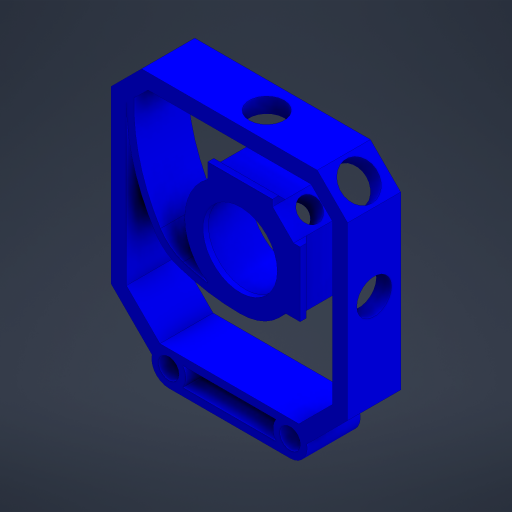
# Autodesk Inventor part: Half Inch Lense Holder (V5)
Saved by Autodesk Inventor 2023.4 (Build 274418000, 418)
## iProperties
Created: 2022-07-25
Part Number: Half Inch Lense Holder (V5)
Material: Generic
Document SubType Name: Modeling
Designer: xSibe
Density: 1 g/cm^3
Appearance: Plastic Blue
Author: xSibe
Autodesk Inventor part; units mm, degrees
ref_plane "YZ Plane" through (0, 0, 0) normal (1, 0, 0) x (0, 1, 0)
ref_plane "XZ Plane" through (0, 0, 0) normal (0, 1, 0) x (-1, 0, 0)
sketch "Sketch1" plane through (0, 0, 0) normal (0, 0, 1) x (1, 0, 0)
  circle A0 centre (10, 3.85) radius 1.5625 projected
  circle A1 centre (-10, 3.85) radius 1.5625 projected
  line L0 (-16.9, 0) -> (16.9, 0) projected
  line L1 (16.9, 0) -> (16.9, 7.7) projected
  line L2 (-16.9, 7.7) -> (16.9, 7.7) projected
  line L3 (-16.9, 0) -> (-16.9, 7.7) projected
  circle A2 centre (-10, 3.85) radius 2.8125
  circle A3 centre (10, 3.85) radius 2.8125
  line L4 (-10, 6.6625) -> (10, 6.6625)
  line L5 (10, 1.0375) -> (-10, 1.0375)
  line L6 (-10, 2.2875) -> (10, 2.2875)
  line L7 (-10, 5.4125) -> (10, 5.4125)
  line L8 (-17.05, 7.7) -> (-17.05, 42.1) projected
  line L9 (17.05, 7.7) -> (17.05, 42.1) projected
  line L10 (-17.05, 24.9) -> (17.05, 24.9)
  line L11 (0, 24.9) -> (1.7678, 26.6678)
  line L12 (0, 24.9) -> (2.5, 24.9) construction
  circle A4 centre (1.7678, 26.6678) radius 7
  circle A5 centre (1.7678, 26.6678) radius 6.325
  circle A6 centre (1.7678, 26.6678) radius 9.125
  line L13 (1.7678, 26.6678) -> (1.7678, 35.7928)
  line L14 (1.7678, 35.7928) -> (1.7678, 35.2928)
  line L15 (-3.5697, 34.0428) -> (7.1053, 34.0428)
  line L16 (7.1053, 34.0428) -> (7.1053, 36.5428)
  line L17 (7.1053, 36.5428) -> (-3.5697, 36.5428)
  line L18 (-3.5697, 36.5428) -> (-3.5697, 34.0428)
  line L19 (-3.5697, 34.0428) -> (7.1053, 36.5428) construction
  line L20 (7.1053, 34.0428) -> (-3.5697, 36.5428) construction
  line L21 (1.7678, 26.6678) -> (8.2201, 33.1201)
  line L22 (8.2201, 33.1201) -> (7.7782, 32.6782)
  line L23 (10.6066, 31.9711) -> (7.0711, 35.5066)
  line L24 (7.0711, 35.5066) -> (4.9497, 33.3853)
  line L25 (4.9497, 33.3853) -> (8.4853, 29.8497)
  line L26 (8.4853, 29.8497) -> (10.6066, 31.9711)
  line L27 (10.6066, 31.9711) -> (4.9497, 33.3853) construction
  line L28 (7.0711, 35.5066) -> (8.4853, 29.8497) construction
  line L29 (10.6066, 31.9711) -> (15.6066, 31.9711) construction
  line L30 (9.1428, 21.3303) -> (9.1428, 32.0053)
  line L31 (9.1428, 32.0053) -> (11.6428, 32.0053)
  line L32 (11.6428, 32.0053) -> (11.6428, 21.3303)
  line L33 (11.6428, 21.3303) -> (9.1428, 21.3303)
  line L34 (1.7678, 35.7928) -> (1.7678, 37.7928)
  line L35 (11.6428, 26.6678) -> (13.6428, 26.6678)
  line L36 (-10.2178, 5.4322) -> (10.2178, 5.4322)
  line L37 (19.4678, 14.6822) -> (19.4678, 39.3678)
  line L38 (14.4678, 44.3678) -> (-14.4678, 44.3678)
  line L39 (-19.4678, 39.3678) -> (-19.4678, 14.6822)
  line L40 (-19.4678, 5.4322) -> (19.4678, 44.3678) construction
  line L41 (19.4678, 5.4322) -> (-19.4678, 44.3678) construction
  line L42 (-10.2178, 5.4322) -> (-19.4678, 14.6822)
  line L43 (10.2178, 5.4322) -> (19.4678, 14.6822)
  line L44 (14.4678, 44.3678) -> (19.4678, 39.3678)
  line L45 (-14.4678, 44.3678) -> (-19.4678, 39.3678)
  line L46 (-15.5033, 46.8678) -> (-21.9678, 40.4033)
  line L47 (-21.9678, 40.4033) -> (-21.9678, 13.6467)
  line L48 (-21.9678, 13.6467) -> (-11.2533, 2.9322)
  line L49 (-11.2533, 2.9322) -> (11.2533, 2.9322)
  line L50 (11.2533, 2.9322) -> (21.9678, 13.6467)
  line L51 (21.9678, 13.6467) -> (21.9678, 40.4033)
  line L52 (21.9678, 40.4033) -> (15.5033, 46.8678)
  line L53 (15.5033, 46.8678) -> (-15.5033, 46.8678)
  line L54 (-13.4322, 41.8678) -> (-16.9678, 38.3322)
  line L55 (-16.9678, 38.3322) -> (-16.9678, 15.7178)
  line L56 (-16.9678, 15.7178) -> (-9.1822, 7.9322)
  line L57 (-9.1822, 7.9322) -> (9.1822, 7.9322)
  line L58 (9.1822, 7.9322) -> (16.9678, 15.7178)
  line L59 (16.9678, 15.7178) -> (16.9678, 38.3322)
  line L60 (16.9678, 38.3322) -> (13.4322, 41.8678)
  line L61 (13.4322, 41.8678) -> (-13.4322, 41.8678)
  line L62 (16.9678, 15.7178) -> (16.9678, 8.6467)
  line L63 (-16.9678, 15.7178) -> (-16.9678, 12.1822)
  line L64 (-19.4678, 14.6822) -> (-19.4678, 11.1467)
  line L65 (19.4678, 14.6822) -> (19.4678, 11.1467)
  circle A7 centre (-10, 3.85) radius 1.705
  circle A8 centre (10, 3.85) radius 1.707
  line L66 (1.7678, 17.5428) -> (-10.7322, 17.5428)
  line L67 (-10.7322, 17.5428) -> (-10.7322, 20.0428)
  arc A9 (-10.7322, 20.0428) -> (1.7678, 17.5428) centre (1.7678, 50.0428) ccw
  arc A10 (-16.9678, 38.3322) -> (-10.7322, 20.0428) centre (12.9724, 38.3322) ccw
  arc A11 (-9.9438, 21.0703) -> (-3.5428, 19.2473) centre (1.7678, 50.0428) ccw
  arc A12 (-15.6893, 39.6107) -> (-9.9438, 21.0703) centre (12.9724, 38.3322) ccw
  line L68 (-9.9438, 21.0703) -> (-11.3596, 23.1309)
  line L69 (-10.7322, 20.0428) -> (-12.1754, 22.0841)
  arc A13 (-12.1754, 22.0841) -> (-8.418, 19.1802) centre (-6.1815, 25.9568) ccw
  arc A14 (-11.3596, 23.1309) -> (-7.6204, 20.2363) centre (-5.5693, 26.7483) ccw
  line L70 (10, 6.6625) -> (11.448, 6.6625)
  line L71 (-10, 6.6625) -> (-11.448, 6.6625)
  point P0 (0, 0)
  point P1 (-7.6615, 2.2875)
  point P2 (-7.6615, 5.4125)
  point P3 (7.6615, 5.4125)
  point P4 (7.6615, 2.2875)
  point P5 (7.3415, 2.9322)
  point P6 (-7.3415, 2.9322)
  point P7 (-11.1858, 6.4003)
  point P8 (11.1858, 6.4003)
  point P9 (-3.5697, 34.0689)
  point P10 (9.1689, 21.3303)
  point P11 (9.1689, 32.0053)
  point P12 (9.741, 31.1055)
  point P13 (6.2055, 34.641)
  point P14 (7.1053, 34.0689)
  point P15 (12.7519, 4.4308)
  point P16 (-12.7519, 4.4308)
  point P17 (5.6072, 34.0428)
  point P18 (-4.0859, 33.6678)
  point P19 (8.7678, 20.8141)
  point P20 (9.1428, 30.5072)
  point P21 (10.8928, 26.6678)
  point P22 (10.5724, 32.0053)
  point P23 (8.7678, 32.5215)
  point P24 (7.6215, 33.6678)
  point P25 (1.7678, 35.7928)
  point P26 (7.1053, 35.4724)
  point P27 (8.2201, 33.1201)
  point P28 (-17.05, 12.2645)
  point P29 (16.9678, 24.9)
  point P30 (17.05, 12.2645)
  point P31 (-16.9678, 24.9)
  point P32 (16.9678, 12.1822)
  point P33 (10.7199, 24.9)
  point P34 (-7.1844, 24.9)
  point P35 (-17.05, 41.7855)
  point P36 (17.05, 41.7855)
  point P37 (7.6748, 5.4322)
  point P38 (-7.6748, 5.4322)
  point P39 (12.4855, 7.7)
  point P40 (-12.4855, 7.7)
  point P41 (-12.9122, 24.9)
  point P42 (-12.9287, 24.9)
  point P43 (-11.8314, 21.5976)
  point P44 (9.1428, 24.9)
  point P45 (11.6428, 24.9)
  point P46 (-12.3792, 24.9)
  point P47 (-13.7856, 24.9)
  point P48 (-11.0227, 22.6405)
  point P49 (7.0178, 35.4533)
  point P50 (10.5533, 31.9178)
  point P51 (8.7178, 27.5029)
  point P52 (8.5409, 24.9)
  point P53 (-5.0053, 24.9)
  dimension "d0" = 1.25
  dimension "d1" = 1.25
  dimension "d2" = 2.5
  dimension "d3" = 45
  dimension "d4" = 14
  dimension "d5" = 0.675
  dimension "d6" = 2.125
  dimension "d7" = 0.5
  dimension "d8" = 10.675
  dimension "d9" = 2.5
  dimension "d10" = 0.625
  dimension "d11" = 5
  dimension "d12" = 135
  dimension "d13" = 3
  dimension "d14" = 2
  dimension "d15" = 2
  dimension "d16" = 38.9355
  dimension "d17" = 38.9355
  dimension "d18" = 9.25
  dimension "d19" = 9.25
  dimension "d20" = 9.25
  dimension "d21" = 9.25
  dimension "d22" = 5
  dimension "d23" = 5
  dimension "d24" = 5
  dimension "d25" = 5
  dimension "d26" = 2.5
  dimension "d46" = 2.5
  dimension "d48" = 0.1425
  dimension "d49" = 0.1445
  dimension "d50" = 12.5
  dimension "d51" = 2.5
  dimension "d52" = 1.25
  dimension "d53" = 2.5
  dimension "d54" = 2.5
  constraints: 132 end point, 28 point on circle, 19 point on line, 15 tangent, 13 centre point, 13 parallel, 10 midpoint, 8 perpendicular, 7 horizontal, 4 symmetric about line, 2 equal length, 2 vertical, 1 coincident, 15 other
  measures "d0" radial gap between concentric circles of A1 A2
  measures "d1" radial gap between concentric circles of A0 A3
  measures "d2" distance of L11.start L11.end
  measures "d3" angle of L12 L11
  measures "d4" diameter of A4
  measures "d5" radial gap between concentric circles of A4 A5
  measures "d6" radial gap between concentric circles of A4 A6
  measures "d7" distance of L13.end L14.end
  measures "d8" distance of L17.end L16.end
  measures "d9" distance of L16.end L15.end
  measures "d10" distance of L21.end L22.end
  measures "d11" distance of L23.start L23.end
  measures "d12" angle of L29 L23
  measures "d13" distance of L24.end L23.end
  measures "d14" distance of L13.end L34.end
  measures "d15" distance of L35.start L35.end
  measures "d16" distance of L40.end L41.end
  measures "d17" distance of L41.end L40.start
  measures "d18" distance of L36.start L40.start
  measures "d19" distance of L39.end L40.start
  measures "d20" distance of L36.end L41.start
  measures "d21" distance of L37.start L41.start
  measures "d22" distance of L38.start L40.end
  measures "d23" distance of L37.end L40.end
  measures "d24" distance of L38.end L41.end
  measures "d25" distance of L39.start L41.end
  measures "d26" distance between parallel lines of L38 L53
  measures "d46" distance between parallel lines of L38 L61
  measures "d48" radial gap between concentric circles of A1 A7
  measures "d49" radial gap between concentric circles of A0 A8
  measures "d50" distance of L66.start L66.end
  measures "d51" distance of L66.end L67.end
  measures "d52" radial gap between concentric circles of A9 A11
  measures "d53" distance of L68.start L68.end
  measures "d54" distance of L67.end L69.end
extrude "Extrusion1" add sketch "Sketch1" along normal mid plane 8.75 contours A8 L49 A3 L7 | L7 A3 L36 A8 | A8 L43 A3 L50 | L50 A3 L6 A8 | A8 L6 A3 L49 | L7 A2 L36 A3 | L36 A3 L43 A8 | A3 L43 L2 L50 | L36 A2 L4 A3 | L7 A7 L36 A2 | A2 L49 A7 L7 | A3 L5 A2 L6 | A3 L70 L43 | L2 L43 L62 L50 | A2 L6 A7 L49 | L36 A7 L42 A2 | A2 L48 A7 L6 | L62 L43 L9 L50 | A2 L42 L71 | L42 A2 L48 L2 | L2 L48 L8 L42 | L62 L59 L10 L9 L43 | L9 L43 L65 L50 | L42 A7 L48 A2 | L42 L8 L10 L55 L63 | L9 L44 L37 L43 | L48 L64 L42 L8 | L42 L39 L45 L8 | L10 L59 L60 L61 L54 L55 L8 L45 L38 L44 L9 | L32 L33 A6 L10 | L10 A6 L26 L23 L31 L32 | A10 L54 A12 L10 | L10 A12 A11 A6 A9 A13 L69 A10 | A6 L33 L30 L10 | L10 L30 L26 A6 | L30 L33 A6 L10 A4 | L10 A4 L25 L26 L30 | A6 L18 L15 L13 A4 L10 | A14 L68 A12 | L30 L31 A6 L26 | L26 L25 L21 A6 L31 L30 | A6 L31 L23 L26 | L31 A6 L16 L23 | L18 L17 L34 A6 | A6 L13 L15 L18 | L68 A14 A11 | L23 L24 A6 L34 L17 L16 | L16 A6 L24 L23 | L13 L15 L24 L25 A4 | A6 L24 L15 L13 | L25 L24 L15 L16 A6 L21 | L16 L15 L24 A6
sketch "Sketch2" plane through (0, 0, 0) normal (0, 0, 1) x (1, 0, 0)
  circle A0 centre (1.7678, 26.6678) radius 7 projected
  circle A1 centre (1.7678, 26.6678) radius 6.125
  line L0 (12.7519, 4.4308) -> (19.4678, 11.1467) projected
  line L1 (19.4678, 11.1467) -> (19.4678, 39.3678) projected
  line L2 (19.4678, 39.3678) -> (14.4678, 44.3678) projected
  line L3 (14.4678, 44.3678) -> (-14.4678, 44.3678) projected
  line L4 (-14.4678, 44.3678) -> (-19.4678, 39.3678) projected
  line L5 (-19.4678, 39.3678) -> (-19.4678, 11.1467) projected
  line L6 (-19.4678, 11.1467) -> (-12.7519, 4.4308) projected
  arc A2 (-12.7519, 4.4308) -> (-10, 1.0375) centre (-10, 3.85) ccw projected
  line L7 (-10, 1.0375) -> (10, 1.0375) projected
  arc A3 (10, 1.0375) -> (12.7519, 4.4308) centre (10, 3.85) ccw projected
  line L8 (7.1053, 35.4724) -> (7.1053, 36.5428) projected
  line L9 (7.1053, 36.5428) -> (-3.5697, 36.5428) projected
  line L10 (-3.5697, 36.5428) -> (-3.5697, 34.0689) projected
  arc A4 (-3.5697, 34.0689) -> (-3.5428, 19.2473) centre (1.7678, 26.6678) ccw projected
  arc A5 (-7.6204, 20.2363) -> (-3.5428, 19.2473) centre (1.7678, 50.0428) ccw projected
  arc A6 (-11.3596, 23.1309) -> (-7.6204, 20.2363) centre (-5.5693, 26.7483) ccw projected
  arc A7 (-15.6893, 39.6107) -> (-11.3596, 23.1309) centre (12.9724, 38.3322) ccw projected
  line L11 (-15.6893, 39.6107) -> (-13.4322, 41.8678) projected
  line L12 (-13.4322, 41.8678) -> (13.4322, 41.8678) projected
  line L13 (13.4322, 41.8678) -> (16.9678, 38.3322) projected
  line L14 (16.9678, 38.3322) -> (16.9678, 12.1822) projected
  line L15 (16.9678, 12.1822) -> (11.448, 6.6625) projected
  line L16 (-11.448, 6.6625) -> (-16.9678, 12.1822) projected
  line L17 (-16.9678, 12.1822) -> (-16.9678, 38.3322) projected
  arc A8 (-16.9678, 38.3322) -> (-12.1754, 22.0841) centre (12.9724, 38.3322) ccw projected
  line L18 (-12.1754, 22.0841) -> (-11.8314, 21.5976) projected
  arc A9 (-11.8314, 21.5976) -> (-8.418, 19.1802) centre (-6.1815, 25.9568) ccw projected
  arc A10 (-8.418, 19.1802) -> (1.7678, 17.5428) centre (1.7678, 50.0428) ccw projected
  arc A11 (1.7678, 17.5428) -> (9.1689, 21.3303) centre (1.7678, 26.6678) ccw projected
  line L19 (9.1689, 21.3303) -> (11.6428, 21.3303) projected
  line L20 (11.6428, 21.3303) -> (11.6428, 32.0053) projected
  line L21 (11.6428, 32.0053) -> (10.5724, 32.0053) projected
  line L22 (10.5724, 32.0053) -> (7.1053, 35.4724) projected
  arc A12 (7.6615, 5.4125) -> (7.6615, 2.2875) centre (10, 3.85) ccw projected
  arc A13 (-7.6615, 2.2875) -> (-7.6615, 5.4125) centre (-10, 3.85) ccw projected
  line L23 (11.448, 6.6625) -> (-11.448, 6.6625) projected
  line L24 (-7.6615, 5.4125) -> (7.6615, 5.4125) projected
  line L25 (7.6615, 2.2875) -> (-7.6615, 2.2875) projected
  point P0 (0, 0)
  point P1 (8.7678, 26.6678)
  point P2 (8.7678, 26.6678)
  point P3 (8.7678, 26.6678)
  dimension "d30" = 0.875
  constraints: 1 centre point
  measures "d30" radial gap between concentric circles of A0 A1
extrude "Extrusion2" add sketch "Sketch2" against normal blind 0.875 from surface at 4.375 contours A0
sketch "Sketch3" plane through (19.4678, 13.6467, -4.375) normal (1, 0, 0) x (0, 0, -1)
  line L0 (0, 7.6836) -> (-8.75, 7.6836) projected
  line L1 (0, 18.3586) -> (0, 7.6836) projected
  line L2 (0, 18.3586) -> (-8.75, 18.3586) projected
  line L3 (-8.75, 7.6836) -> (-8.75, 18.3586) projected
  line L4 (-4.375, 18.3586) -> (-4.375, 7.6836)
  circle A0 centre (-4.375, 13.0211) radius 2.875
  point P0 (-4.375, -13.6467)
  dimension "d33" = 5.75
  constraints: 3 midpoint, 2 end point, 1 centre point
  measures "d33" diameter of A0
extrude "Extrusion3" cut sketch "Sketch3" against normal up to surface (2.5 mm away) contours A0 L4 | L4 A0
sketch "Sketch4" plane through (10.9865, 32.0053, -4.375) normal (0, 1, 0) x (1, 0, 0)
  line L0 (0.6562, 0) -> (0.6562, -8.75) projected
  line L1 (-0.4141, 0) -> (0.6562, 0) projected
  line L2 (0.6562, -8.75) -> (-0.4141, -8.75) projected
  line L3 (0.6562, -8.75) -> (-0.4141, -8.75)
  line L4 (-0.4141, -8.75) -> (-0.4141, -7.75)
  line L5 (-0.4141, -7.75) -> (0.6562, -7.75)
  line L6 (0.6562, -7.75) -> (0.6562, -8.75)
  line L7 (0.6562, -7.75) -> (-0.4141, -6.6796)
  line L8 (0.6562, -7.75) -> (2.1699, -7.75) construction
  line L9 (-0.4141, -4.375) -> (0.6562, -4.375)
  line L10 (0.6562, -1) -> (-0.4141, -2.0704)
  line L11 (-0.4141, 0) -> (-0.4141, -8.75) projected
  point P0 (-10.9865, -4.375)
  point P1 (0.6562, -1)
  point P2 (0.6562, -7.75)
  point P3 (0.6562, -7.75)
  point P4 (-0.4141, -7.75)
  dimension "d36" = 1
  dimension "d37" = 135
  constraints: 16 end point, 3 horizontal, 2 midpoint, 2 parallel, 2 symmetric about line, 1 equal length, 1 perpendicular, 1 point on line
  measures "d36" distance of L2.end L4.end
  measures "d37" angle of L8 L7
extrude "Extrusion4" cut sketch "Sketch4" against normal up to surface (10.675 mm away) contours L0 L9 L11 L10 | L0 L7 L11 L9
ref_plane "Work Plane1" through (11.6428, 36.5428, 4.375) normal (0.7071068, -0.7071068, 0) x (0, 0, -1)
mirror "Mirror1" about plane through (11.6428, 36.5428, 4.375) normal (0.7071068, -0.7071068, 0) of "Extrusion3", "Extrusion4"
sketch "Sketch5" plane through (20.2, 38.6355, 4.375) normal (0.7071068, 0.7071068, 0) x (0.7071068, -0.7071068, 0)
  line L0 (-7.0227, 8.75) -> (-2.1194, 8.75) projected
  line L1 (-2.1194, 0) -> (-7.0227, 0) projected
  circle A0 centre (-4.5711, 4.375) radius 1.875
  line L2 (-7.0711, 4.375) -> (-2.0711, 4.375)
  circle A1 centre (-4.5711, 4.375) radius 3
  line L3 (-2.1194, 6.6796) -> (-2.1194, 2.0704) projected
  line L4 (-7.0227, 2.0704) -> (-7.0227, 6.6796) projected
  line L5 (-2.1194, 8.75) -> (-2.1194, 6.6796) projected
  line L6 (-7.0227, 6.6796) -> (-7.0227, 8.75) projected
  line L7 (-7.0227, 0) -> (-7.0227, 2.0704) projected
  line L8 (-2.1194, 2.0704) -> (-2.1194, 0) projected
  point P0 (13.0359, 4.375)
  dimension "d40" = 3.75
  dimension "d41" = 6
  constraints: 2 centre point, 2 end point, 1 coincident, 1 midpoint
  measures "d40" diameter of A0
  measures "d41" diameter of A1
extrude "Extrusion5" cut sketch "Sketch5" against normal blind 5 contours L4 A1 | A1 L3 L2 A0 L4 | A1 L3 | L4 L2 A0 L3 A1 | L2 A0 | A0 L2
extrude "Extrusion6" cut sketch "Sketch5" against normal up to next from surface at -11.496 contours L2 A0 | A0 L2
equation "\"d19\" = d18"
equation "\"d20\" = d18"
equation "\"d21\" = d20"
equation "\"d23\" = d22"
equation "\"d24\" = d22"
equation "\"d25\" = d24"
body "Solid1"
